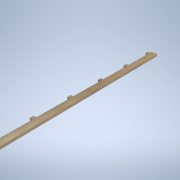
# Autodesk Inventor part: steun
Saved by Autodesk Inventor 2021 (Build 250183000, 183)
## iProperties
Created: 2021-03-16
Part Number: steun
Material: Wood (Maple)
Document SubType Name: Modeling
Designer: ZiweZhang
Density: 0.67 g/cm^3
Appearance: Natural Maple - Glossy Dark Tint
Author: ZiweZhang
Autodesk Inventor part; units mm, degrees
ref_plane "YZ Plane" through (0, 0, 0) normal (1, 0, 0) x (0, 1, 0)
ref_plane "XZ Plane" through (0, 0, 0) normal (0, 1, 0) x (-1, 0, 0)
ref_plane "XY Plane" through (0, 0, 0) normal (0, 0, 1) x (1, 0, 0)
sketch "Sketch1" plane through (0, 0, 0) normal (0, 1, 0) x (-1, 0, 0)
  line L0 (-5, 3.5) -> (-5, -3.5)
  line L1 (-5, -3.5) -> (2, -3.5)
  line L2 (5, -0.5) -> (5, 3.5)
  line L3 (5, 3.5) -> (2, 3.5)
  line L4 (5, -0.5) -> (2, -0.5)
  line L5 (2, -0.5) -> (2, -3.5)
  line L6 (5, 37.5) -> (2, 37.5)
  line L7 (5, 37.5) -> (5, 41.5)
  line L8 (5, 41.5) -> (2, 41.5)
  line L9 (5, 75.5) -> (2, 75.5)
  line L10 (5, 75.5) -> (5, 79.5)
  line L11 (5, 79.5) -> (2, 79.5)
  line L12 (5, 113.5) -> (2, 113.5)
  line L13 (5, 113.5) -> (5, 117.5)
  line L14 (5, 117.5) -> (2, 117.5)
  line L15 (5, 151.5) -> (2, 151.5)
  line L16 (5, 151.5) -> (5, 155.5)
  line L17 (5, 155.5) -> (2, 155.5)
  line L18 (5, 189.5) -> (2, 189.5)
  line L19 (5, 189.5) -> (5, 193.5)
  line L20 (5, 193.5) -> (2, 193.5)
  line L21 (2, 3.5) -> (2, 37.5)
  line L22 (2, 41.5) -> (2, 75.5)
  line L23 (2, 79.5) -> (2, 113.5)
  line L24 (2, 117.5) -> (2, 151.5)
  line L25 (2, 155.5) -> (2, 189.5)
  line L26 (-5, 193.5) -> (-5, 3.5)
  line L27 (2, 193.5) -> (-5, 193.5)
  point P0 (0, 0)
  dimension "d10" = 3
  dimension "d18" = 38
  constraints: 56 end point, 5 collinear, 3 vertical, 2 parallel, 2 perpendicular, 1 horizontal, 1 point on line, 34 other
  measures "d10" distance of L2.start L4.end
  measures "d18" distance of L2.start L6.start
extrude "Extrusion1" add sketch "Sketch1" along normal blind 3
body "Solid1"
